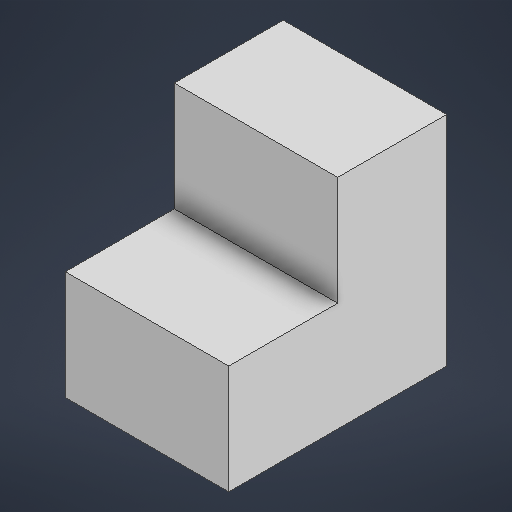
# Autodesk Inventor part: iso
Saved by Autodesk Inventor 2025.1 (Build 291241000, 241)
## iProperties
Created: 2025-06-16
Part Number: iso
Material: Generic
Document SubType Name: Modeling
Designer: riters
Density: 1 g/cm^3
Appearance: Default
Author: riters
Autodesk Inventor part; units mm, degrees
ref_plane "YZ Plane" through (0, 0, 0) normal (1, 0, 0) x (0, 1, 0)
ref_plane "XZ Plane" through (0, 0, 0) normal (0, 1, 0) x (-1, 0, 0)
ref_plane "XY Plane" through (0, 0, 0) normal (0, 0, 1) x (1, 0, 0)
sketch "Sketch1" plane through (0, 0, 0) normal (1, 0, 0) x (0, 1, 0)
  line L0 (-12.7, 12.7) -> (0, 12.7)
  line L1 (12.7, 0) -> (12.7, -12.7)
  line L2 (12.7, -12.7) -> (-12.7, -12.7)
  line L3 (-12.7, -12.7) -> (-12.7, 12.7)
  line L4 (-12.7, 12.7) -> (12.7, -12.7) construction
  line L5 (0, 0) -> (-12.7, -12.7) construction
  line L6 (0, 0) -> (12.7, 0)
  line L7 (0, 12.7) -> (0, 0)
  line L8 (12.7, 0) -> (0, 0)
  dimension "d0" = 25.4
  constraints: 18 end point, 2 horizontal, 2 midpoint, 2 parallel, 2 perpendicular, 1 collinear, 1 point on line, 1 vertical
  measures "d0" distance of L1.end L2.end
extrude "Extrusion1" add sketch "Sketch1" along normal mid plane 19.05
body "Solid1"
